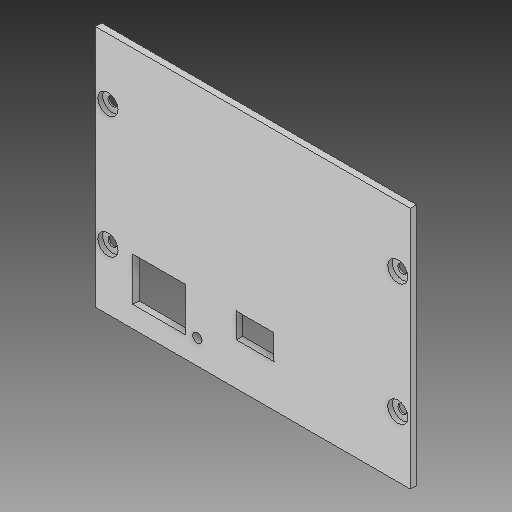
# Autodesk Inventor part: Ra-Manager_Painel-Placas
Saved by Autodesk Inventor 2019.4 (Build 234330000, 330)
## iProperties
Created: 2020-03-12
Part Number: Ra-Manager_Painel-Placas
Material: Aço, carbono
Document SubType Name: Modeling
Designer: caio.santos
Density: 7.85 g/cm^3
Appearance: Padrão
Author: caio.santos
Autodesk Inventor part; units mm, degrees
ref_plane "YZ Plane" through (0, 0, 0) normal (1, 0, 0) x (0, 1, 0)
ref_plane "XZ Plane" through (0, 0, 0) normal (0, 1, 0) x (-1, 0, 0)
ref_plane "XY Plane" through (0, 0, 0) normal (0, 0, 1) x (1, 0, 0)
sketch "Esboço1" plane through (0, 0, 0) normal (0, 0, 1) x (1, 0, 0)
  line L0 (-50.5, 39) -> (50.5, 39)
  line L1 (50.5, 39) -> (50.5, -39)
  line L2 (50.5, -39) -> (-50.5, -39)
  line L3 (-50.5, -39) -> (-50.5, 39)
  point P0 (0, 0)
  dimension "d2" = 101
  dimension "d3" = 78
  dimension "d4" = 101
  dimension "d5" = 50.5
  dimension "d6" = 39
  constraints: 8 end point, 2 perpendicular, 1 horizontal
  measures "d2" distance of L0.start L0.end
  measures "d3" distance of L0.end L1.end
  measures "d4" distance of L1.end L2.end
  measures "d5" distance from line of point (0, 0) L1
  measures "d6" distance from line of point (0, 0) L0
extrude "Extrusão1" add sketch "Esboço1" against normal blind 2
sketch "Esboço2" plane through (0, 0, 0) normal (0, 0, 1) x (1, 0, 0)
  line L0 (50.5, -39) -> (-50.5, -39) projected
  line L1 (42.5, 39) -> (42.5, -39) construction
  line L2 (-50.5, -39) -> (-50.5, 39) projected
  line L3 (50.5, 39) -> (50.5, -39) projected
  line L4 (-42.5, 39) -> (-42.5, -39) construction
  line L5 (-50.5, 39) -> (50.5, 39) projected
  line L6 (-50.5, 19.5) -> (50.5, 19.5) construction
  line L7 (-50.5, -19.5) -> (50.5, -19.5) construction
  line L8 (-50.5, 39) -> (50.5, 39) projected
  line L9 (-46.5, 39) -> (-46.5, -39) construction
  line L10 (50.5, -39) -> (-50.5, -39) projected
  line L11 (46.5, 39) -> (46.5, -39) construction
  point P0 (0, 0)
  point P1 (-46.5, 19.5)
  point P2 (-46.5, -19.5)
  point P3 (46.5, -19.5)
  point P4 (46.5, 19.5)
  dimension "d32" = 8
  dimension "d33" = 8
  dimension "d34" = 4
  dimension "d35" = 4
  dimension "d36" = 19.5
  dimension "d37" = 58.5
  dimension "d38" = 78
  dimension "d39" = 78
  constraints: 18 point on line, 12 end point, 6 perpendicular
  measures "d32" distance between parallel lines of L1 L3
  measures "d33" distance between parallel lines of L2 L4
  measures "d34" distance of L2.end L9.start
  measures "d35" distance of L3.start L11.start
  measures "d36" distance between parallel lines of L5 L6
  measures "d37" distance between parallel lines of L5 L7
  measures "d38" distance from line of L1.start L0
  measures "d39" distance from line of L4.start L0
hole "Furo2" at (-46.5, 19.5, 0) at (-46.5, -19.5, 0) at (46.5, -19.5, 0) at (46.5, 19.5, 0) direction (0, 0, -1) diameter 3 end through all counterbore diameter 6.5 counterbore depth 1.5
sketch "Esboço3" plane through (0, 0, 0) normal (0, 0, 1) x (1, 0, 0)
  line L0 (-22.0376, -18.7161) -> (-38.0376, -18.7161) projected
  line L1 (-38.0376, -18.7161) -> (-38.0376, -31.7161) projected
  line L2 (-22.0376, -31.7161) -> (-22.0376, -18.7161) projected
  line L3 (-38.0376, -31.7161) -> (-22.0376, -31.7161) projected
  line L4 (-39.6791, -31.6586) -> (39.7959, -31.6586) projected
  line L5 (-18.3542, -30.6586) -> (-17.2542, -30.6586) projected
  line L6 (-18.8542, -30.6586) -> (-18.3542, -30.6586) projected
  line L7 (-17.2542, -30.6586) -> (-16.7542, -30.6586) projected
  line L8 (-16.5542, -30.6586) -> (-16.7542, -30.6586) projected
  line L9 (-16.5542, -30.6586) -> (-16.5542, -30.6586) projected
  line L10 (-16.5542, -31.6586) -> (-16.5542, -30.6586) projected
  line L11 (-16.6542, -31.6586) -> (-16.5542, -31.6586) projected
  line L12 (-16.6542, -31.6586) -> (-17.0042, -31.6586) projected
  line L13 (-17.1042, -31.6586) -> (-17.0042, -31.6586) projected
  line L14 (-17.1042, -31.6586) -> (-17.6542, -31.6586) projected
  line L15 (-17.9542, -31.6586) -> (-17.6542, -31.6586) projected
  line L16 (-17.9542, -31.6586) -> (-18.9542, -31.6586) projected
  line L17 (-19.0542, -31.6586) -> (-18.7042, -31.6586) projected
  line L18 (-19.0542, -30.6586) -> (-19.0542, -31.6586) projected
  line L19 (-9.5679, -25.4931) -> (-14.5971, -25.4931) projected
  line L20 (12.8419, -25.4356) -> (10.7613, -25.4356) projected
  line L21 (10.7613, -31.6586) -> (10.7613, -25.4356) projected
  line L22 (12.8419, -29.4261) -> (12.8419, -28.4101) projected
  line L23 (-14.5971, -31.7161) -> (-14.5971, -25.4931) projected
  line L24 (-9.5679, -31.7161) -> (-9.5679, -25.4931) projected
  line L25 (-21.5376, -32.2161) -> (-38.5376, -32.2161)
  line L26 (-38.5376, -32.2161) -> (-38.5376, -18.2161)
  line L27 (-38.5376, -18.2161) -> (-21.5376, -18.2161)
  line L28 (-21.5376, -18.2161) -> (-21.5376, -32.2161)
  circle A0 centre (-17.8042, -31.1586) radius 1.5
  line L29 (-9.5679, -25.4356) -> (10.7613, -25.4356) construction
  line L30 (-5.2876, -25.4356) -> (6.7124, -25.4356)
  line L31 (-5.2876, -25.4356) -> (-5.2876, -17.4356)
  line L32 (-5.2876, -17.4356) -> (6.7124, -17.4356)
  line L33 (6.7124, -17.4356) -> (6.7124, -25.4356)
  point P0 (0, 0)
  point P1 (39.7959, -31.6586)
  dimension "d49" = 17
  dimension "d50" = 14
  dimension "d51" = 17
  dimension "d52" = 3
  dimension "d61" = 8
  dimension "d70" = 0.5
  dimension "d71" = 0
  dimension "d72" = 0.5
  dimension "d74" = 12
  dimension "d75" = 16.25
  constraints: 16 end point, 3 perpendicular, 2 vertical, 1 centre point, 1 horizontal, 6 other
  measures "d49" distance of L25.start L25.end
  measures "d50" distance of L25.end L26.end
  measures "d51" distance of L26.end L27.end
  measures "d52" diameter of A0
  measures "d61" distance of L30.start L31.end
  measures "d70" distance between parallel lines of L26 L1
  measures "d71" distance of A0.centre point (-17.804, -31.159)
  measures "d72" distance between parallel lines of L0 L27
  measures "d74" distance of L31.end L32.end
  measures "d75" distance from line of L28 L30.start
extrude "Extrusão2" cut sketch "Esboço3" against normal blind 10 contours L2 L4 L1 L0 | L0 L1 L4 L26 L27 L28 L2 | L4 L28 L25 L26 L1 L3 L2 | L2 L3 L1 L4 | L4 A0 | L4 A0 | L31 L32 L33 L30
equation "\"d2\" = 2 * d5"
equation "\"d3\" = 2 * d6"
equation "\"d4\" = d2"
equation "\"d33\" = d32"
equation "\"d34\" = d35"
equation "\"d35\" = 0.5 * d32"
